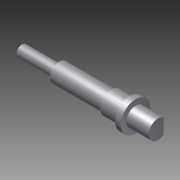
# Autodesk Inventor part: 13_1087_015
Saved by Autodesk Inventor 2014 (Build 180170000, 170)
## iProperties
Created: 2013-09-02
Part Number: 13_1087_015
Material: Allgemein
Document SubType Name: Modeling
Designer: vogel
Density: 1 g/cm^3
Appearance: Vorgabe
Author: vogel
Autodesk Inventor part; units mm, degrees
ref_plane "YZ Plane" through (0, 0, 0) normal (1, 0, 0) x (0, 1, 0)
ref_plane "XZ Plane" through (0, 0, 0) normal (0, 1, 0) x (-1, 0, 0)
ref_plane "XY Plane" through (0, 0, 0) normal (0, 0, 1) x (1, 0, 0)
sketch "Skizze1" plane through (0, 0, 0) normal (0, 0, 1) x (1, 0, 0)
  line L0 (-55.7318, 0) -> (9.2886, 0) projected
  line L1 (0, -0.8) -> (0, 4.8) projected
  line L2 (0, 0) -> (0, 2.5)
  line L3 (0, 0) -> (-46.4431, 0)
  line L4 (0, 2.5) -> (-6, 2.5)
  line L5 (-6, 2.5) -> (-6, 3)
  line L6 (-7.5, 3) -> (-13.5, 3)
  line L7 (-13.5, 3) -> (-13.5, 2.5)
  line L8 (-13.5, 2.5) -> (-26.5, 2.5)
  line L9 (-26.5, 2.5) -> (-26.5, 1.5)
  line L10 (-26.5, 1.5) -> (-36.5, 1.5)
  line L11 (-36.5, 1.5) -> (-36.5, 0)
  line L12 (-36.5, 0) -> (0, 0)
  line L13 (-6, 3) -> (-6, 4)
  line L14 (-6, 4) -> (-7.5, 4)
  line L15 (-7.5, 4) -> (-7.5, 3)
  dimension "d0" = 5
  dimension "d1" = 6
  dimension "d4" = 5
  dimension "d5" = 13
  dimension "d6" = 3
  dimension "d7" = 10
  dimension "d9" = 8
  dimension "d10" = 1.5
  dimension "d11" = 7.5
  dimension "d15" = 6
  constraints: 28 end point, 9 perpendicular, 3 point on line, 2 parallel, 1 collinear
  measures "d0" diameter of L4 L3
  measures "d1" diameter of L6 L3
  measures "d4" diameter of L8 L3
  measures "d5" distance of L7.end L8.end
  measures "d6" diameter of L10 L3
  measures "d7" distance of L9.end L10.end
  measures "d9" diameter of L14 L3
  measures "d10" distance of L13.end L14.end
  measures "d11" distance between parallel lines of L15 L2
  measures "d15" distance from line of L7.end L15
revolve "Umdrehung1" add sketch "Skizze1" angle 360 about axis through (0, 0, 0) along (-1, 0, 0)
sketch "Skizze2" plane through (0, 0, 0) normal (1, 0, 0) x (0, 0, -1)
  circle A0 centre (0, 0) radius 2.5 projected
  line L0 (0, -5.6) -> (0, 5.6) projected
  line L1 (5.6, 0) -> (-5.6, 0) projected
  line L2 (-2, 1.5) -> (2, 1.5)
  dimension "d12" = 1.5
  constraints: 2 end point, 2 point on circle, 1 parallel
  measures "d12" distance between parallel lines of L2 L1
extrude "Extrusion1" cut sketch "Skizze2" against normal blind 4 contours L2 L0 A0 | L0 L2 A0
